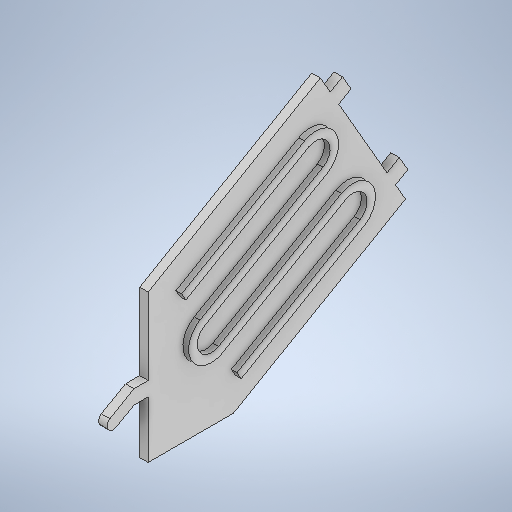
# Autodesk Inventor part: autour hélice autre côté
Saved by Autodesk Inventor 2026.2 (Build 302298010, 298A)
## iProperties
Created: 2026-04-02
Part Number: autour hélice autre côté
Material: Générique
Document SubType Name: Modeling
Designer: Genon
Density: 1 g/cm^3
Appearance: Par défaut
Author: Genon
Autodesk Inventor part; units mm, degrees
ref_plane "YZ Plane" through (0, 0, 0) normal (1, 0, 0) x (0, 1, 0)
ref_plane "XZ Plane" through (0, 0, 0) normal (0, 1, 0) x (-1, 0, 0)
ref_plane "Plan de construction1" through (0, 0, 0) normal (0, 0.5, -0.8660254) x (1, 0, 0)
sketch "Esquisse1" plane through (0, 0, 0) normal (0, 0.5, -0.8660254) x (1, 0, 0)
  line L0 (-40, 0) -> (-40, -30)
  line L1 (-40, -30) -> (-37, -30)
  line L2 (-40, -30) -> (-37, -30)
  line L3 (-37, -30) -> (-37, 30)
  line L4 (-37, 30) -> (-40, 30)
  line L5 (-40, 30) -> (-40, -30)
  point P0 (0, 0)
  point P1 (-37, 0)
  point P2 (-37, -30)
  dimension "d2" = 30
  dimension "d3" = 3
  dimension "d4" = 60
  dimension "d49" = 37
  dimension "d50" = 40
  constraints: 12 end point, 2 horizontal, 2 midpoint, 2 parallel, 1 perpendicular, 1 vertical
  measures "d2" distance of L0.start L0.end
  measures "d3" distance of L0.end L1.end
  measures "d4" distance of L3.end L2.end
  measures "d49" distance of point (0, 0) point (-37, 0)
  measures "d50" distance of point (0, 0) point (-40, 0)
extrude "Extrusion1" add sketch "Esquisse1" along normal blind 70
ref_plane "Plan de construction2" through (0, 0, 15) normal (0, 0, 1) x (1, 0, 0)
sketch "Esquisse2" plane through (0, 0, 15) normal (0, 0, 1) x (1, 0, 0)
  line L0 (-40, -25.9808) -> (-40, 25.9808) projected
  line L1 (-37, 25.9808) -> (-37, -25.9808) projected
  line L2 (-40, 25.9808) -> (-37, 25.9808) projected
  line L3 (-37, -25.9808) -> (-40, -25.9808) projected
  line L4 (-37, 60.9808) -> (-37, 9.0192) projected
  line L5 (-40, 25.9808) -> (-37, 25.9808)
  line L6 (-37, 25.9808) -> (-37, 35.9808)
  line L7 (-37, 35.9808) -> (-40, 35.9808)
  line L8 (-40, 35.9808) -> (-40, 25.9808)
  point P0 (0, 0)
  point P1 (37, 25.9808)
  dimension "d46" = 10
  constraints: 8 end point, 2 parallel, 1 horizontal, 1 perpendicular, 1 point on line
  measures "d46" distance of L6.end L5.end
extrude "Extrusion2" add sketch "Esquisse2" against normal blind 30 contours L0 L2 L1 L3
ref_plane "Plan de construction3" through (-37, -25.9808, 15) normal (1, 0, 0) x (0, 0, -1)
sketch "Esquisse3" plane through (-37, -25.9808, 15) normal (1, 0, 0) x (0, 0, -1)
  line L0 (0, 0) -> (0, 20)
  line L1 (0, 51.9615) -> (0, 0) projected
  line L2 (0, 20) -> (-5, 20)
  line L3 (-5, 20) -> (-5, 25)
  line L4 (-5, 25) -> (0, 25)
  point P0 (15, 25.9808)
  dimension "d16" = 20
  dimension "d17" = 5
  constraints: 8 end point, 2 perpendicular, 2 point on line, 1 vertical
  measures "d16" distance of L0.start L0.end
  measures "d17" distance of L0.end L2.end
extrude "Extrusion3" add sketch "Esquisse3" against normal up to surface (3 mm away)
ref_plane "Plan de construction6" through (0, -11.0705, 19.1747) normal (0, 0.5, -0.8660254) x (1, 0, 0)
sketch "Esquisse5" plane through (0, -11.0705, 19.1747) normal (0, 0.5, -0.8660254) x (1, 0, 0)
  line L0 (-40, -9.1506) -> (-40, -4.8205) projected
  line L1 (-37, -9.1506) -> (-40, -9.1506) projected
  line L2 (-37, -4.8205) -> (-40, -4.8205) projected
  line L3 (-37, -9.1506) -> (-37, -4.8205) projected
  point P0 (0, 0)
extrude "Extrusion5" add sketch "Esquisse5" along normal mid plane 15
fillet "Congé1" radius 2 2 edges at (-38.5, -6.8958, 30.2452) (-38.5, -10.6458, 28.0801)
sketch "Esquisse12" plane through (-37, -25.9808, 15) normal (1, 0, 0) x (0, 0, -1)
  line L0 (0, 25) -> (-1.3397, 25) projected
  line L1 (0, 25) -> (-6.1432, 25)
  line L2 (-6.1432, 25) -> (-6.1432, 29.4942)
  line L3 (-6.1432, 29.4942) -> (0, 29.4942)
  line L4 (0, 29.4942) -> (0, 25)
  point P0 (15, 25.9808)
  constraints: 8 end point, 2 parallel, 1 horizontal, 1 perpendicular
extrude "Extrusion11" cut sketch "Esquisse12" against normal through all
sketch "Esquisse13" plane through (0, 35, -60.6218) normal (0, 0.5, -0.8660254) x (-1, 0, 0)
  line L0 (37, 30) -> (37, -30) projected
  line L1 (37, 0) -> (37, 20)
  line L2 (37, 20) -> (40, 20)
  line L3 (40, -30) -> (40, 30) projected
  line L4 (40, 20) -> (40, 23)
  line L5 (40, 23) -> (37, 23)
  line L6 (37, 23) -> (37, 17)
  line L7 (37, 17) -> (40, 17)
  line L8 (40, 17) -> (40, 20)
  line L9 (37, 0) -> (37, -20)
  line L10 (37, -20) -> (40, -20)
  line L11 (40, -20) -> (40, -17)
  line L12 (40, -17) -> (37, -17)
  line L13 (37, -17) -> (37, -23)
  line L14 (37, -23) -> (40, -23)
  line L15 (40, -23) -> (40, -20)
  point P0 (0, 0)
  point P1 (37, 23)
  point P2 (37, 17)
  point P3 (40, 17)
  dimension "d53" = 20
  dimension "d54" = 3
  dimension "d55" = 6
  dimension "d56" = 20
  dimension "d57" = 3
  dimension "d58" = 6
  constraints: 28 end point, 11 point on line, 8 perpendicular, 1 collinear, 1 midpoint
  measures "d53" distance of L1.start L1.end
  measures "d54" distance of L2.end L4.end
  measures "d55" distance of L5.end L6.end
  measures "d56" distance of L1.start L9.end
  measures "d57" distance of L10.end L11.end
  measures "d58" distance of L12.end L13.end
extrude "Extrusion12" add sketch "Esquisse13" along normal blind 5 contours L5 L3 L2 L0 | L2 L3 L7 L0 | L12 L3 L10 L0 | L10 L3 L14 L0
sketch "Esquisse14" plane through (-37, -25.9808, 15) normal (1, 0, 0) x (0, 0, -1)
  line L0 (11.2627, 44.9296) -> (54.564, 69.9296)
  line L1 (11.2627, 44.9296) -> (61.2627, 44.9296) construction
  arc A0 (59.564, 61.2694) -> (54.564, 69.9296) centre (57.064, 65.5995) ccw
  line L2 (59.564, 61.2694) -> (16.2401, 36.3085)
  line L3 (26.3922, 19.4858) -> (76.3922, 19.4858) construction
  line L4 (11.2627, 44.9296) -> (9.7627, 47.5277)
  line L5 (9.7627, 47.5277) -> (53.064, 72.5277)
  line L6 (59.564, 61.2694) -> (61.064, 58.6713)
  line L7 (61.064, 58.6713) -> (17.7627, 33.6713)
  line L8 (17.7627, 33.6713) -> (22.7627, 25.011)
  line L9 (17.7627, 33.6713) -> (27.7627, 33.6713) construction
  line L10 (22.7627, 25.011) -> (66.064, 50.011)
  line L11 (17.7627, 33.6713) -> (22.7627, 25.011)
  arc A1 (17.7627, 33.6713) -> (22.7627, 25.011) centre (20.2627, 29.3412) ccw
  line L12 (22.7627, 25.011) -> (24.2627, 22.413)
  line L13 (24.2627, 22.413) -> (67.564, 47.413)
  arc A2 (16.2401, 36.3085) -> (24.2853, 22.3738) centre (20.2627, 29.3412) ccw
  arc A3 (61.064, 58.6713) -> (53.064, 72.5277) centre (57.064, 65.5995) ccw
  line L14 (67.564, 47.413) -> (72.564, 38.7527)
  line L15 (67.564, 47.413) -> (77.564, 47.413) construction
  line L16 (72.564, 38.7527) -> (29.2627, 13.7527)
  line L17 (29.2627, 13.7527) -> (30.7627, 11.1546)
  line L18 (30.7627, 11.1546) -> (74.064, 36.1546)
  arc A4 (72.564, 38.7527) -> (67.564, 47.413) centre (70.064, 43.0828) ccw
  arc A5 (74.064, 36.1546) -> (66.064, 50.011) centre (70.064, 43.0828) ccw
  line L19 (16.2401, 36.3085) -> (17.7627, 33.6713)
  line L20 (22.7627, 25.011) -> (24.2853, 22.3738)
  line L21 (59.564, 61.2694) -> (61.064, 58.6713)
  dimension "d61" = 50
  dimension "d62" = 30
  dimension "d63" = 10
  dimension "d64" = 5
  dimension "d71" = 3
  dimension "d72" = 3
  dimension "d75" = 10
  dimension "d76" = 60
  dimension "d78" = 90
  dimension "d79" = 3
  dimension "d80" = 10
  dimension "d81" = 60
  dimension "d82" = 50
  dimension "d83" = 90
  dimension "d84" = 3
  dimension "d85" = 5
  constraints: 44 end point, 13 point on circle, 7 perpendicular, 6 centre point, 5 point on line, 4 horizontal, 3 coincident, 3 collinear, 3 equal length, 2 tangent
  measures "d61" distance of L0.start L0.end
  measures "d62" angle of L1 L0
  measures "d63" distance of L0.end L2.start
  measures "d64" radius of A0
  measures "d71" distance of L0.start L4.end
  measures "d72" distance of L2.start L6.end
  measures "d75" distance of L7.end L8.end
  measures "d76" angle of L8 L9
  measures "d78" angle of L10 L8
  measures "d79" distance of L8.end L12.end
  measures "d80" distance of L13.end L14.end
  measures "d81" angle of L14 L15
  measures "d82" distance of L14.end L16.end
  measures "d83" angle of L14 L16
  measures "d84" distance of L16.end L17.end
  measures "d85" radius of A4
extrude "Extrusion13" add sketch "Esquisse14" along normal blind 2 contours L4 L5 A3 L6 A0 L0 | L6 L7 L19 L2 | L19 A1 L12 L20 A2 | L12 L10 A5 L18 L17 L16 A4 L13
